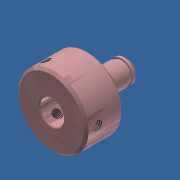
# Autodesk Inventor part: None_Magnet_Extender_Split_Top
Saved by Autodesk Inventor 2015 (Build 190159000, 159)
## iProperties
Created: 2015-01-06
Part Number: None_Magnet_Extender_Split_Top
Material: Aluminum 6061
Document SubType Name: Modeling
Designer: ice
Mass: 1.63117 g
Surface Area: 7.28726 cm^2
Volume: 0.604135 cm^3
Density: 2.7 g/cm^3
Appearance: Aluminum - Flat
Author: ice
Autodesk Inventor part; units mm, degrees
sketch "Sketch1" plane through (0, 0, 0) normal (1, 0, 0) x (0, 1, 0)
  line L0 (32, 0) -> (32, 2.45)
  line L1 (32, 2.45) -> (30.5, 2.45)
  line L2 (30.5, 2.45) -> (30.5, 2.125)
  line L3 (30.5, 2.125) -> (29.7, 2.125)
  line L4 (29.7, 2.125) -> (29.7, 2.45)
  line L5 (29.7, 2.45) -> (26.7, 2.45)
  line L6 (26.7, 2.45) -> (26.7, 2.125)
  line L7 (26.7, 2.125) -> (25.9, 2.125)
  line L8 (25.9, 2.125) -> (25.9, 2.45)
  line L9 (25.9, 2.45) -> (24.4, 2.45)
  line L10 (23.4, 2.5) -> (24.4, 2.5)
  line L11 (24.4, 2.5) -> (24.4, 2.45)
  line L12 (23.4, 2.5) -> (23.4, 7.5)
  line L13 (32, 2.45) -> (31, 2.45)
  line L14 (32, 2.45) -> (32, 1.45)
  line L15 (23.4, 7.5) -> (15.4, 7.5)
  line L16 (15.4, 7.5) -> (15.4, 0)
  line L17 (32, 0) -> (15.4, 0)
  point P0 (0, 0)
  dimension "d345" = 1.5
  dimension "d346" = 0.325
  dimension "d347" = 0.8
  dimension "d348" = 3
  dimension "d349" = 0.325
  dimension "d350" = 0.8
  dimension "d353" = 1
  dimension "d354" = 1
  dimension "d355" = 1
  dimension "d401" = 8
  dimension "d402" = 16.6
  constraints: 36 end point, 7 perpendicular, 5 horizontal, 3 point on line, 1 vertical
  measures "d345" distance of L0.end L1.end
  measures "d346" distance of L1.end L2.end
  measures "d347" distance of L2.end L3.end
  measures "d348" distance of L4.end L5.end
  measures "d349" distance of L5.end L6.end
  measures "d350" distance of L6.end L7.end
  measures "d353" distance of L10.start L10.end
  measures "d354" distance of L0.end L13.end
  measures "d355" distance of L0.end L14.end
  measures "d401" distance of L12.end L15.end
  measures "d402" distance of L16.end L0.start
revolve "Revolution1" add sketch "Sketch1" angle 360 about axis through (0, 32, 0) along (0, -1, 0)
chamfer "Chamfer8" distance 1 angle 45 1 edges at (0, 32, -2.45)
sketch "Sketch13" plane through (0, 32, 0) normal (0, 1, 0) x (1, 0, 0)
  circle A0 centre (0, 0) radius 1
  point P0 (0, 0)
  dimension "d359" = 2
  constraints: 1 centre point, 1 coincident
  measures "d359" diameter of A0
hole "Hole10" at (0, 32, 0) direction (0, -1, 0) diameter 2 end through all
ref_plane "Work Plane8" through (0, 26.3, 0) normal (0, 1, 0) x (1, 0, 0)
ref_plane "Work Plane9" through (0, 30.1, 0) normal (0, 1, 0) x (1, 0, 0)
sketch "Sketch16" plane through (0, 15.4, 0) normal (0, -1, 0) x (1, 0, 0)
  circle A0 centre (0, 0) radius 2.55
  dimension "d404" = 5.1
  constraints: 1 centre point, 1 coincident
  measures "d404" diameter of A0
hole "Hole12" at (0, 15.4, 0) direction (0, 1, 0) diameter 5.1 depth 5
sketch "Sketch19" plane through (0, 15.4, 0) normal (0, -1, 0) x (1, 0, 0)
  circle A0 centre (0, 0) radius 7.5 projected
  line L0 (0, 0) -> (7.5, 0)
  line L1 (0, 0) -> (-3.75, -6.4952)
  line L2 (0, 0) -> (7.5, 0) construction
  line L3 (0, 0) -> (-3.75, 6.4952)
  line L4 (0, 0) -> (7.5, 0) construction
  point P0 (0, 0)
  dimension "d423" = 7.5
  dimension "d424" = 120
  dimension "d425" = 7.5
  dimension "d426" = 120
  constraints: 10 end point, 3 horizontal, 2 equal length, 1 horizontal alignment, 1 other
  measures "d423" distance of L0.start L1.end
  measures "d424" angle of L1 L2
  measures "d425" distance of L0.start L3.end
  measures "d426" angle of L4 L3
ref_plane "Work Plane12" through (7.5, 15.4, 0) normal (1, 0, 0) x (0, 1, 0)
ref_plane "Work Plane13" through (-3.75, 15.4, 6.4952) normal (-0.5, 0, 0.866) x (0, -1, 0)
ref_plane "Work Plane14" through (-3.75, 15.4, -6.4952) normal (-0.5, 0, -0.866) x (0, -1, 0)
sketch "Sketch20" plane through (-3.75, 15.4, -6.4952) normal (-0.5, 0, -0.866) x (0, -1, 0)
  line L0 (0, -7.5) -> (0, 7.5) projected
  line L1 (0, 0) -> (-2.5, 0)
  point P0 (15.4, 0)
  dimension "d427" = 2.5
  constraints: 2 end point, 1 horizontal, 1 midpoint
  measures "d427" distance of L1.start L1.end
sketch "Sketch21" plane through (-3.75, 15.4, 6.4952) normal (-0.5, 0, 0.866) x (0, -1, 0)
  line L0 (0, -7.5) -> (0, 7.5) projected
  line L1 (0, 0) -> (-2.5, 0)
  point P0 (15.4, 0)
  dimension "d428" = 2.5
  constraints: 2 end point, 1 horizontal, 1 midpoint
  measures "d428" distance of L1.start L1.end
sketch "Sketch22" plane through (7.5, 15.4, 0) normal (1, 0, 0) x (0, 1, 0)
  line L0 (0, 0) -> (2.5, 0)
  point P0 (-15.4, 0)
  dimension "d429" = 2.5
  constraints: 2 end point, 1 horizontal
  measures "d429" distance of L0.start L0.end
hole "Hole14" at (-3.75, 17.9, 6.4952) direction (0.5, 0, -0.866) diameter 1.9 depth 6
hole "Hole15" at (-3.75, 17.9, -6.4952) direction (0.5, 0, 0.866) diameter 1.9 depth 6
hole "Hole16" at (7.5, 17.9, 0) direction (-1, 0, 0) diameter 1.9 depth 6
thread "Thread25" size "M2x0.4" class "6H" standard "ANSI Metric M Profile" full length
thread "Thread26" size "M2x0.4" class "6H" standard "ANSI Metric M Profile" full length
thread "Thread27" size "M2x0.4" class "6H" standard "ANSI Metric M Profile" full length
chamfer "Chamfer9" distance 0.5 angle 45 2 edges at (0, 23.4, -7.5) (0, 15.4, -7.5)
chamfer "Chamfer10" distance 0.2 angle 45 1 edges at (0, 15.4, 2.55)
ref_plane "Work Plane15" through (-1.25, 15.4, 2.1651) normal (-0.5, 0, 0.866) x (0, -1, 0)
ref_plane "Work Plane16" through (2.5, 15.4, 0) normal (1, 0, 0) x (0, 1, 0)
ref_plane "Work Plane17" through (-1.25, 15.4, -2.1651) normal (-0.5, 0, -0.866) x (0, -1, 0)
body "Solid1"
